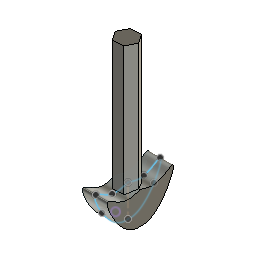
horse_support (Autodesk Fusion 360 design; units mm, degrees)
part number: 2026-05-20-21-49-29-160
Autodesk Fusion 360 part; units mm, degrees
derive "DerivedContext1"
sketch "Sketch1" plane through (0, 0, 0) normal (1, 0, 0) x (0, 1, 0)
  line L0 (-161.6595, 88.3093) -> (-161.6595, 78.1224)
  spline S0 degree 5 poles (-161.6595, 88.3093) (-161.4963, 88.2786) (-161.1532, 88.2007) (-160.5882, 88.034) (-159.7352, 87.7468) (-158.5139, 87.4576) (-157.166, 87.4242) (-155.7427, 87.767) (-154.3291, 88.4385) (-153.036, 89.236) (-151.9779, 89.8931) (-151.2551, 90.1487) (-150.9341, 89.8224) (-151.0266, 88.8948) (-151.5022, 87.4675) (-152.3028, 85.7161) (-153.3565, 83.8482) (-154.59, 82.0593) (-155.9416, 80.4924) (-157.3598, 79.2495) (-158.8043, 78.3979) (-159.9575, 78.0617) (-160.8129, 78.0126) (-161.3782, 78.0707) (-161.6595, 78.1224) knots 0 0 0 0 0 0 0.05 0.1 0.15 0.2 0.25 0.3 0.35 0.4 0.45 0.5 0.55 0.6 0.65 0.7 0.75 0.8 0.85 0.9 0.95 1 1 1 1 1 1
  line L1 (-165.3917, 89.0107) -> (-157.9274, 87.6079)
  line L2 (-157.7822, 77.4094) -> (-165.5368, 78.8354)
  spline S1 degree 5 poles (-161.6595, 88.3093) (-161.8227, 88.2786) (-162.1659, 88.2007) (-162.7308, 88.034) (-163.5838, 87.7468) (-164.8051, 87.4576) (-166.153, 87.4242) (-167.5763, 87.767) (-168.9899, 88.4385) (-170.283, 89.236) (-171.3411, 89.8931) (-172.064, 90.1487) (-172.3849, 89.8224) (-172.2924, 88.8948) (-171.8169, 87.4675) (-171.0162, 85.7161) (-169.9626, 83.8482) (-168.729, 82.0593) (-167.3775, 80.4924) (-165.9592, 79.2495) (-164.5147, 78.3979) (-163.3616, 78.0617) (-162.5061, 78.0126) (-161.9409, 78.0707) (-161.6595, 78.1224) knots 0 0 0 0 0 0 0.05 0.1 0.15 0.2 0.25 0.3 0.35 0.4 0.45 0.5 0.55 0.6 0.65 0.7 0.75 0.8 0.85 0.9 0.95 1 1 1 1 1 1
  line L3 (-157.9274, 89.0107) -> (-165.3917, 87.6079)
  line L4 (-165.5368, 77.4094) -> (-157.7822, 78.8354)
  point P0 (-156.5652, 87.6135)
  point P1 (-151.319, 90)
  point P2 (-153.319, 84)
  point P3 (-166.7538, 87.6135)
  point P4 (-172, 90)
  point P5 (-170, 84)
  constraint vertical L0
  constraint coincident L0 S0.end
  constraint midpoint L0.start L1
  constraint midpoint L0.end L2
  constraint symmetric P0 L0 P3
  constraint symmetric P1 L0 P4
  constraint symmetric P2 L0 P5
  constraint symmetric L0 S0.start S1.start
  constraint symmetric L0 S0.end S1.end
  constraint symmetric L0 L1.start L3.start
  constraint symmetric L0 L1.end L3.end
  constraint symmetric L0 L2.start L4.start
  constraint symmetric L0 L2.end L4.end
extrude "Extrude1" add sketch "Sketch1" along normal mid plane 8
sketch "Sketch2" plane through (-4, 0, 0) normal (-1, 0, 0) x (0, -1, 0)
  spline S0 degree 5 poles (161.6595, 78.1224) (161.9409, 78.0707) (162.5061, 78.0126) (163.3616, 78.0617) (164.5147, 78.3979) (165.9592, 79.2495) (167.3775, 80.4924) (168.729, 82.0593) (169.9626, 83.8482) (171.0162, 85.7161) (171.8169, 87.4675) (172.2924, 88.8948) (172.3849, 89.8224) (172.064, 90.1487) (171.3411, 89.8931) (170.283, 89.236) (168.9899, 88.4385) (167.5763, 87.767) (166.153, 87.4242) (164.8051, 87.4576) (163.5838, 87.7468) (162.7308, 88.034) (162.1659, 88.2007) (161.8227, 88.2786) (161.6595, 88.3093) knots -1 -1 -1 -1 -1 -1 -0.95 -0.9 -0.85 -0.8 -0.75 -0.7 -0.65 -0.6 -0.55 -0.5 -0.45 -0.4 -0.35 -0.3 -0.25 -0.2 -0.15 -0.1 -0.05 0 0 0 0 0 0
  spline S1 degree 5 poles (161.6595, 88.3093) (161.4963, 88.2786) (161.1532, 88.2007) (160.5882, 88.034) (159.7352, 87.7468) (158.5139, 87.4576) (157.166, 87.4242) (155.7427, 87.767) (154.3291, 88.4385) (153.036, 89.236) (151.9779, 89.8931) (151.2551, 90.1487) (150.9341, 89.8224) (151.0266, 88.8948) (151.5022, 87.4675) (152.3028, 85.7161) (153.3565, 83.8482) (154.59, 82.0593) (155.9416, 80.4924) (157.3598, 79.2495) (158.8043, 78.3979) (159.9575, 78.0617) (160.8129, 78.0126) (161.3782, 78.0707) (161.6595, 78.1224) knots 0 0 0 0 0 0 0.05 0.1 0.15 0.2 0.25 0.3 0.35 0.4 0.45 0.5 0.55 0.6 0.65 0.7 0.75 0.8 0.85 0.9 0.95 1 1 1 1 1 1
ref_plane "WorkPlane1" through (-4, -160.339, 88.8588) normal (0, 0, 1) x (-1, 0, 0)
sketch "Sketch3" plane through (0, 0, 88.8588) normal (0, 0, 1) x (1, 0, 0)
  line L0 (1.9423, -164.9116) -> (3.4927, -161.7737)
  line L1 (3.4927, -161.7737) -> (1.5503, -158.8621)
  line L2 (1.5503, -158.8621) -> (-1.9423, -159.0884)
  line L3 (-1.9423, -159.0884) -> (-3.4927, -162.2263)
  line L4 (-3.4927, -162.2263) -> (-1.5503, -165.1379)
  line L5 (-1.5503, -165.1379) -> (1.9423, -164.9116)
  point P0 (0, -162)
  dimension "d4" = 3.5
  measures "d4" distance of L0.start P0
extrude "Extrude2" add sketch "Sketch3" along normal blind 40 and the other way blind 1.5
